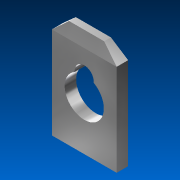
# Autodesk Inventor part: Soanar Power Module Pin D
Saved by Autodesk Inventor 2016 (Build 200138000, 138)
## iProperties
Created: 2013-08-06
Material: Nickel-Copper Alloy 400
Document SubType Name: Modeling
Designer: sdarley
Density: 8.83 g/cm^3
Appearance: Chrome - Polished
Project: Power Entry Module - Soanar PP4003
Description: Soanar Power Module Pin D
Author: sdarley
Title: Soanar Power Module Pin D
Revision Number: 1
Autodesk Inventor part; units mm, degrees
ref_plane "YZ Plane" through (0, 0, 0) normal (1, 0, 0) x (0, 1, 0)
ref_plane "XZ Plane" through (0, 0, 0) normal (0, 1, 0) x (-1, 0, 0)
ref_plane "XY Plane" through (0, 0, 0) normal (0, 0, 1) x (1, 0, 0)
sketch "Sketch1" plane through (0, 0, 0) normal (0, 1, 0) x (-1, 0, 0)
  line L0 (-2.4, 0) -> (2.4, 0)
  line L1 (2.4, 0) -> (2.4, 7.8)
  line L2 (2.4, 7.8) -> (-2.4, 7.8)
  line L3 (-2.4, 7.8) -> (-2.4, 0)
  arc A0 (-0.7, 4.9198) -> (0.7, 4.9198) centre (0, 3.65) ccw
  arc A1 (0.7, 4.9198) -> (-0.7, 4.9198) centre (0, 4.9959) ccw
  point P0 (0, 0)
  point P1 (0, 7.8)
  point P2 (0, 0)
  dimension "d0" = 4.8
  dimension "d1" = 7.8
  dimension "d2" = 5.6
  dimension "d3" = 1.45
  dimension "d4" = 2.1
  dimension "d5" = 1.4
  constraints: 8 end point, 4 point on circle, 2 centre point, 2 midpoint, 2 parallel, 2 vertical alignment, 1 coincident, 1 horizontal, 1 perpendicular
  measures "d0" distance between parallel lines of L1 L3
  measures "d1" distance between parallel lines of L0 L2
  measures "d3" radius of A0
  measures "d4" distance edge to line of A1 L2
  measures "d5" distance of A0.end A0.start
extrude "Extrusion1" add sketch "Sketch1" along normal mid plane 0.85
chamfer "Chamfer1" distance 1.1 distance2 1 1 edges at (2.4, 0, 7.8) measured on face at (-0.8, -0.1417, 7.8)
chamfer "Chamfer2" distance 1.1 distance2 1 1 edges at (-2.4, 0, 7.8) measured on face at (0.0667, 0.1417, 7.8)
chamfer "Chamfer3" distance 1 distance2 0.175 1 edges at (0, 0.425, 7.8) measured on face at (0, 0.425, 0.7333)
chamfer "Chamfer4" distance 1 distance2 0.175 1 edges at (0, -0.425, 7.8) measured on face at (0, -0.425, 0.7333)
body "Solid1"
